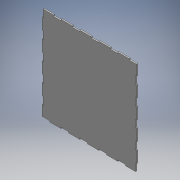
# Autodesk Inventor part: Bbase
Saved by Autodesk Inventor 2016 (Build 200138000, 138)
## iProperties
Created: 2016-12-11
Part Number: Bbase
Material: Generic
Document SubType Name: Modeling
Designer: NacostaMobile
Density: 1 g/cm^3
Appearance: Default
Author: NacostaMobile
Autodesk Inventor part; units mm, degrees
ref_plane "YZ Plane" through (0, 0, 0) normal (1, 0, 0) x (0, 1, 0)
ref_plane "XZ Plane" through (0, 0, 0) normal (0, 1, 0) x (-1, 0, 0)
ref_plane "XY Plane" through (0, 0, 0) normal (0, 0, 1) x (1, 0, 0)
sketch "Sketch1" plane through (0, 0, 0) normal (0, 1, 0) x (-1, 0, 0)
  line L0 (247, 0) -> (247, -20)
  line L1 (247, -20) -> (250, -20)
  line L2 (247, -50) -> (247, -70)
  line L3 (247, -70) -> (250, -70)
  line L4 (247, -50) -> (250, -50)
  line L5 (250, -20) -> (250, -50)
  line L6 (247, -100) -> (247, -120)
  line L7 (247, -150) -> (247, -170)
  line L8 (247, -200) -> (247, -220)
  line L9 (247, -220) -> (250, -220)
  line L10 (247, -200) -> (250, -200)
  line L11 (247, -170) -> (250, -170)
  line L12 (247, -150) -> (250, -150)
  line L13 (247, -120) -> (250, -120)
  line L14 (247, -100) -> (250, -100)
  line L15 (250, -220) -> (250, -247)
  line L16 (250, -170) -> (250, -200)
  line L17 (250, -70) -> (250, -100)
  line L18 (250, -120) -> (250, -150)
  line L19 (3, -250) -> (3, -230)
  line L20 (3, -230) -> (0, -230)
  line L21 (3, -200) -> (3, -180)
  line L22 (3, -180) -> (0, -180)
  line L23 (3, -200) -> (0, -200)
  line L24 (0, -230) -> (0, -200)
  line L25 (3, -150) -> (3, -130)
  line L26 (3, -100) -> (3, -80)
  line L27 (3, -50) -> (3, -30)
  line L28 (3, -30) -> (0, -30)
  line L29 (3, -50) -> (0, -50)
  line L30 (3, -80) -> (0, -80)
  line L31 (3, -100) -> (0, -100)
  line L32 (3, -130) -> (0, -130)
  line L33 (3, -150) -> (0, -150)
  line L34 (0, -30) -> (0, -3)
  line L35 (0, -80) -> (0, -50)
  line L36 (0, -180) -> (0, -150)
  line L37 (0, -130) -> (0, -100)
  line L38 (130, -247) -> (150, -247)
  line L39 (150, -250) -> (150, -247)
  line L40 (150, -250) -> (180, -250)
  line L41 (180, -250) -> (180, -247)
  line L42 (200, -250) -> (200, -247)
  line L43 (180, -247) -> (200, -247)
  line L44 (200, -250) -> (230, -250)
  line L45 (230, -250) -> (230, -247)
  line L46 (230, -247) -> (250, -247)
  line L47 (3, -250) -> (30, -250)
  line L48 (30, -250) -> (30, -247)
  line L49 (130, -250) -> (130, -247)
  line L50 (100, -250) -> (130, -250)
  line L51 (100, -250) -> (100, -247)
  line L52 (80, -247) -> (100, -247)
  line L53 (80, -250) -> (80, -247)
  line L54 (50, -250) -> (80, -250)
  line L55 (50, -250) -> (50, -247)
  line L56 (30, -247) -> (50, -247)
  line L57 (230, -250) -> (200, -250)
  line L58 (180, -250) -> (150, -250)
  line L59 (130, -250) -> (100, -250)
  line L60 (80, -250) -> (50, -250)
  line L61 (30, -250) -> (3, -250)
  line L62 (0, -3) -> (20, -3)
  line L63 (20, -3) -> (20, 0)
  line L64 (50, 0) -> (50, -3)
  line L65 (50, -3) -> (70, -3)
  line L66 (70, -3) -> (70, 0)
  line L67 (100, -3) -> (100, 0)
  line L68 (100, -3) -> (120, -3)
  line L69 (120, -3) -> (120, 0)
  line L70 (150, 0) -> (150, -3)
  line L71 (150, -3) -> (170, -3)
  line L72 (170, -3) -> (170, 0)
  line L73 (200, 0) -> (200, 0)
  line L74 (200, 0) -> (200, -3)
  line L75 (200, -3) -> (220, -3)
  line L76 (220, -3) -> (220, 0)
  line L77 (220, 0) -> (247, 0)
  line L78 (170, 0) -> (200, 0)
  line L79 (120, 0) -> (150, 0)
  line L80 (20, 0) -> (50, 0)
  line L81 (70, 0) -> (100, 0)
  point P0 (0, 0)
  dimension "d11" = 20
  dimension "d12" = 20
  dimension "d13" = 20
  dimension "d14" = 20
  dimension "d15" = 20
  dimension "d16" = 20
  dimension "d17" = 20
  dimension "d18" = 20
  dimension "d19" = 30
  dimension "d20" = 30
  dimension "d21" = 30
  dimension "d22" = 30
  dimension "d27" = 20
  dimension "d28" = 3
  dimension "d30" = 20
  dimension "d31" = 3
  dimension "d32" = 20
  dimension "d33" = 20
  dimension "d34" = 3
  dimension "d35" = 20
  dimension "d36" = 3
  dimension "d37" = 20
  dimension "d38" = 30
  dimension "d39" = 30
  dimension "d40" = 250
  dimension "d41" = 20
  dimension "d42" = 20
  dimension "d43" = 20
  dimension "d44" = 20
  dimension "d45" = 20
  dimension "d46" = 20
  dimension "d47" = 27
  constraints: 164 end point, 135 perpendicular, 48 parallel, 7 horizontal, 5 point on line, 5 vertical
  measures "d11" distance of L2.start L2.end
  measures "d12" distance of L6.start L6.end
  measures "d13" distance of L7.start L7.end
  measures "d14" distance of L8.start L8.end
  measures "d15" distance of L21.start L22.start
  measures "d16" distance of L25.start L32.start
  measures "d17" distance of L31.start L26.end
  measures "d18" distance of L29.start L27.end
  measures "d19" distance of L54.start L53.start
  measures "d20" distance of L50.start L50.end
  measures "d21" distance of L39.start L40.end
  measures "d22" distance of L44.end L42.start
  measures "d27" distance from line of L19.start L20
  measures "d28" distance of L20.end L19.end
  measures "d30" distance of L34.end L62.end
  measures "d31" distance of L64.start L64.end
  measures "d32" distance of L64.end L65.end
  measures "d33" distance of L67.start L68.end
  measures "d34" distance of L70.start L70.end
  measures "d35" distance of L70.end L71.end
  measures "d36" distance of L73.end L74.end
  measures "d37" distance of L74.end L75.end
  measures "d38" horizontal distance of L76.end L1.end
  measures "d39" vertical distance of L44.end L9.end
  measures "d40" horizontal distance of L15.end L20.end
  measures "d41" distance of L15.end L45.end
  measures "d42" distance of L41.end L43.end
  measures "d43" distance of L0.start L0.end
  measures "d44" distance of L49.end L38.end
  measures "d45" distance of L53.end L51.end
  measures "d46" distance of L48.end L55.end
  measures "d47" distance of L19.start L48.start
extrude "Extrusion1" add sketch "Sketch1" along normal blind 3
body "Solid1"
